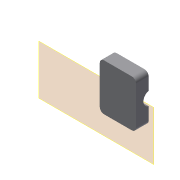
# Autodesk Inventor part: 20_Cube_Insert_Template_magnetic_clamp_v3
Saved by Autodesk Inventor 2022 (Build 260153000, 153)
## iProperties
Created: 2022-01-10
Part Number: 20_Cube_Insert_Template_magnetic_clamp_v3
Material: Generisch
Document SubType Name: Modeling
Designer: diederichbenedict
Density: 1 g/cm^3
Appearance: Vorgabe
Author: diederichbenedict
Autodesk Inventor part; units mm, degrees
ref_plane "YZ Plane" through (0, 0, 0) normal (1, 0, 0) x (0, 1, 0)
ref_plane "XZ Plane" through (0, 0, 0) normal (0, 1, 0) x (-1, 0, 0)
ref_plane "XY Plane" through (0, 0, 0) normal (0, 0, 1) x (1, 0, 0)
ref_plane "Arbeitsebene1" through (0, 0, 0) normal (0, 0, 1) x (1, 0, 0)
sketch "Skizze1" plane through (0, 0, 0) normal (0, 0, 1) x (1, 0, 0)
  circle A0 centre (34.3329, 7.5) radius 3.25 construction
  circle A1 centre (44.3329, 7.5) radius 3.25 construction
  circle A2 centre (34.3329, -7.5) radius 3.25 construction
  circle A3 centre (44.3329, -7.5) radius 3.25 construction
  line L0 (34.3329, 7.5) -> (44.3329, 7.5) construction
  line L1 (44.3329, 7.5) -> (44.3329, -7.5) construction
  line L2 (44.3329, -7.5) -> (34.3329, -7.5) construction
  line L3 (34.3329, -7.5) -> (34.3329, 7.5) construction
  line L4 (47.9329, 11.1) -> (30.7329, 11.1)
  line L5 (30.7329, 11.1) -> (30.7329, -11.1)
  line L6 (30.7329, -11.1) -> (47.9329, -11.1)
  line L7 (47.9329, -11.1) -> (47.9329, 11.1)
  circle A4 centre (34.3329, 7.5) radius 2.5
  circle A5 centre (44.3329, 7.5) radius 2.5
  circle A6 centre (34.3329, -7.5) radius 2.5
  circle A7 centre (44.3329, -7.5) radius 2.5
  point P0 (0, 0)
  dimension "d0" = 3.6
  dimension "d1" = 5
  dimension "d2" = 5
  dimension "d3" = 5
  dimension "d4" = 5
  constraints: 16 end point, 4 centre point, 4 coincident, 4 parallel, 2 perpendicular, 1 horizontal, 3 other
  measures "d0" distance between parallel lines of L0 L4
  measures "d1" diameter of A4
  measures "d2" diameter of A5
  measures "d3" diameter of A6
  measures "d4" diameter of A7
extrude "Extrusion1" add sketch "Skizze1" along normal blind 4
sketch "Skizze2" plane through (0, 0, 4) normal (0, 0, 1) x (1, 0, 0)
  line L0 (30.7329, 11.1) -> (30.7329, -11.1) projected
  line L1 (30.7329, -11.1) -> (47.9329, -11.1) projected
  line L2 (47.9329, -11.1) -> (47.9329, 11.1) projected
  line L3 (47.9329, 11.1) -> (30.7329, 11.1) projected
  circle A0 centre (34.3329, 7.5) radius 2.5 projected
  circle A1 centre (44.3329, 7.5) radius 2.5 projected
  circle A2 centre (34.3329, -7.5) radius 2.5 projected
  circle A3 centre (44.3329, -7.5) radius 2.5 projected
  point P0 (0, 0)
extrude "Extrusion2" add sketch "Skizze2" along normal blind 2 contours L3 L2 L1 L0 | A0 | A1 | A2 | A3
sketch "Skizze3" plane through (47.9329, -11.1, 0) normal (1, 0, 0) x (0, 0, -1)
  circle A0 centre (0, 11.1) radius 3.22 projected
  circle A1 centre (0.7362, 11.1) radius 3.22
  point P0 (0, 11.1)
  dimension "d9" = 6.44
  dimension "d10" = 6.44
  constraints: 1 centre point
  measures "d9" diameter of A0
  measures "d10" diameter of A1
extrude "Extrusion3" cut sketch "Skizze3" against normal through all contours A0 A1 | A0 A1 picked at (-0.5511, 10.842) picked at (3.403, 11.6139)
fillet "Rundung1" radius 2 4 edges at (47.9329, -11.1, 3) (47.9329, 11.1, 3) (30.7329, 11.1, 3) (30.7329, -11.1, 3)
equation "\"d10\" = d9"
